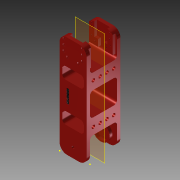
# Autodesk Inventor part: 150mm Link
Saved by Autodesk Inventor 2015 (Build 190159000, 159)
## iProperties
Created: 2016-11-30
Part Number: 150mm Link
Material: Generic
Document SubType Name: Modeling
Designer: Rudge-Top
Density: 1 g/cm^3
Appearance: Orange-Red
Author: Rudge-Top
Autodesk Inventor part; units mm, degrees
ref_plane "YZ Plane" through (0, 0, 0) normal (1, 0, 0) x (0, 1, 0)
ref_plane "XZ Plane" through (0, 0, 0) normal (0, 1, 0) x (-1, 0, 0)
ref_plane "XY Plane" through (0, 0, 0) normal (0, 0, 1) x (1, 0, 0)
sketch "Sketch1" plane through (0, 0, 0) normal (1, 0, 0) x (0, 1, 0)
  line L0 (120, 0) -> (150, 0)
  line L1 (150, 0) -> (150, -40)
  line L2 (150, -40) -> (120, -40)
  line L3 (150, 5) -> (0, 5)
  line L4 (0, -45) -> (150, -45)
  line L5 (150, 0) -> (150, 5)
  line L6 (150, -40) -> (150, -45)
  line L7 (0, -40) -> (0, -45)
  line L8 (0, 0) -> (0, 5)
  line L9 (115, -5) -> (115, -35)
  arc A0 (120, 0) -> (115, -5) centre (120, -5) ccw
  arc A1 (115, -35) -> (120, -40) centre (120, -35) ccw
  line L10 (87.5, 0) -> (62.5, 0)
  line L11 (57.5, -5) -> (57.5, -35)
  line L12 (62.5, -40) -> (87.5, -40)
  line L13 (92.5, -35) -> (92.5, -5)
  arc A2 (87.5, -40) -> (92.5, -35) centre (87.5, -35) ccw
  arc A3 (57.5, -35) -> (62.5, -40) centre (62.5, -35) ccw
  arc A4 (62.5, 0) -> (57.5, -5) centre (62.5, -5) ccw
  arc A5 (92.5, -5) -> (87.5, 0) centre (87.5, -5) ccw
  line L14 (0, 0) -> (30, 0)
  line L15 (35, -5) -> (35, -35)
  line L16 (30, -40) -> (0, -40)
  arc A6 (35, -5) -> (30, 0) centre (30, -5) ccw
  arc A7 (30, -40) -> (35, -35) centre (30, -35) ccw
  point P0 (57.5, -40)
  point P1 (92.5, -40)
  point P2 (35, 0)
  dimension "d1" = 150
  dimension "d2" = 40
  dimension "d3" = 90
  dimension "d4" = 5
  dimension "d5" = 35
  dimension "d6" = 5
  dimension "d7" = 35
  dimension "d8" = 5
  dimension "d9" = 22.5
  dimension "d10" = 5
  dimension "d11" = 35
  dimension "d12" = 5
  constraints: 34 end point, 16 point on circle, 16 tangent, 9 point on line, 8 centre point, 8 perpendicular, 5 equal radius, 3 horizontal, 2 parallel
  measures "d1" distance of L8.start L0.end
  measures "d2" distance of L0.end L1.end
  measures "d3" angle of L0 L1
  measures "d4" distance between parallel lines of L0 L3
  measures "d5" distance between parallel lines of L1 L9
  measures "d6" radius of A0
  measures "d7" distance of point (92.5, -40) point (57.5, -40)
  measures "d8" distance between parallel lines of L3 L10
  measures "d9" distance between parallel lines of L13 L9
  measures "d10" radius of A2
  measures "d11" distance of L8.start point (35, 0)
  measures "d12" radius of A6
extrude "Extrusion1" add sketch "Sketch1" along normal blind 40 contours A0 L9 A1 L2 L6 L4 L7 L16 A7 L15 A6 L14 L8 L3 L5 L0
sketch "Sketch2" plane through (40, 0, 0) normal (1, 0, 0) x (0, 0, -1)
  arc A0 (35, 57.5) -> (40, 62.5) centre (35, 62.5) ccw projected
  line L0 (35, 57.5) -> (5, 57.5) projected
  arc A1 (0, 62.5) -> (5, 57.5) centre (5, 62.5) ccw projected
  line L1 (0, 62.5) -> (0, 87.5) projected
  arc A2 (5, 92.5) -> (0, 87.5) centre (5, 87.5) ccw projected
  line L2 (5, 92.5) -> (35, 92.5) projected
  arc A3 (40, 87.5) -> (35, 92.5) centre (35, 87.5) ccw projected
  line L3 (40, 87.5) -> (40, 62.5) projected
  line L4 (0, 0) -> (0, 30) projected
  arc A4 (5, 35) -> (0, 30) centre (5, 30) ccw projected
  line L5 (5, 35) -> (35, 35) projected
  arc A5 (40, 30) -> (35, 35) centre (35, 30) ccw projected
  line L6 (40, 30) -> (40, 0) projected
  line L7 (40, 0) -> (45, 0) projected
  line L8 (45, 0) -> (45, 150) projected
  line L9 (45, 150) -> (40, 150) projected
  line L10 (40, 150) -> (40, 120) projected
  arc A6 (35, 115) -> (40, 120) centre (35, 120) ccw projected
  line L11 (35, 115) -> (5, 115) projected
  arc A7 (0, 120) -> (5, 115) centre (5, 120) ccw projected
  line L12 (0, 120) -> (0, 150) projected
  line L13 (0, 150) -> (-5, 150) projected
  line L14 (-5, 150) -> (-5, 0) projected
  line L15 (-5, 0) -> (0, 0) projected
  circle A8 centre (35, 45.25) radius 2.5
  circle A9 centre (25, 45.25) radius 2.5
  circle A10 centre (15, 45.25) radius 2.5
  circle A11 centre (5, 45.25) radius 2.5
  circle A12 centre (35, 104.75) radius 2.5
  circle A13 centre (25, 104.75) radius 2.5
  circle A14 centre (15, 104.75) radius 2.5
  circle A15 centre (5, 104.75) radius 2.5
  dimension "d15" = 5
  dimension "d16" = 5
  dimension "d17" = 5
  dimension "d18" = 5
  dimension "d19" = 10
  dimension "d20" = 20
  dimension "d21" = 30
  dimension "d22" = 40
  dimension "d23" = 5
  dimension "d24" = 5
  dimension "d25" = 5
  dimension "d26" = 5
  dimension "d27" = 12.25
  dimension "d28" = 12.25
  dimension "d29" = 12.25
  dimension "d30" = 12.25
  dimension "d31" = 12.25
  dimension "d32" = 12.25
  dimension "d33" = 12.25
  dimension "d34" = 12.25
  constraints: 8 centre point
  measures "d15" diameter of A8
  measures "d16" diameter of A9
  measures "d17" diameter of A10
  measures "d18" diameter of A11
  measures "d19" distance from line of L14 A11.centre
  measures "d20" distance from line of A10.centre L14
  measures "d21" distance from line of A9.centre L14
  measures "d22" distance from line of A8.centre L14
  measures "d23" diameter of A12
  measures "d24" diameter of A13
  measures "d25" diameter of A14
  measures "d26" diameter of A15
  measures "d27" distance from line of A12.centre L2
  measures "d28" distance from line of L2 A13.centre
  measures "d29" distance from line of L2 A14.centre
  measures "d30" distance from line of L2 A15.centre
  measures "d31" distance from line of A8.centre L0
  measures "d32" distance from line of A9.centre L0
  measures "d33" distance from line of A10.centre L0
  measures "d34" distance from line of A11.centre L0
extrude "Extrusion2" cut sketch "Sketch2" against normal blind 25 contours A8 | A9 | A10 | A11 | A12 | A13 | A14 | A15
fillet "Fillet1" radius 11 8 edges at (40, 0, 2.5) (0, 0, 2.5) (40, 0, -42.5) (0, 0, -42.5) (40, 150, 2.5) (40, 150, -42.5) (0, 150, -42.5) (0, 150, 2.5)
sketch "Sketch3" plane through (0, 11, -45) normal (0, 0, -1) x (-1, 0, 0)
  line L0 (0, 51.5) -> (-40, 51.5) projected
  arc A0 (0, 128) -> (-11, 139) centre (-11, 128) ccw projected
  line L1 (-11, 139) -> (-29, 139) projected
  arc A1 (-29, 139) -> (-40, 128) centre (-29, 128) ccw projected
  line L2 (-40, 0) -> (-40, 128) projected
  arc A2 (-40, 0) -> (-29, -11) centre (-29, 0) ccw projected
  line L3 (-11, -11) -> (-29, -11) projected
  arc A3 (-11, -11) -> (0, 0) centre (-11, 0) ccw projected
  line L4 (0, 0) -> (0, 128) projected
  line L5 (-40, 51.5) -> (-40, 46.5) projected
  line L6 (-40, 46.5) -> (-40, 51.5) projected
  line L7 (-40, 51.5) -> (-40, 76.5) projected
  line L8 (-40, 76.5) -> (-40, 81.5) projected
  line L9 (-40, 81.5) -> (-40, 76.5) projected
  line L10 (-40, 76.5) -> (-40, 51.5) projected
  line L11 (-40, 91.25) -> (-40, 96.25) projected
  line L12 (-40, 91.25) -> (-40, 96.25) projected
  line L13 (-40, 31.75) -> (-40, 36.75) projected
  line L14 (-40, 31.75) -> (-40, 36.75) projected
  line L15 (-40, 31.75) -> (-40, 36.75) projected
  line L16 (-40, 31.75) -> (-40, 36.75) projected
  line L17 (-40, 91.25) -> (-40, 96.25) projected
  line L18 (-40, 91.25) -> (-40, 96.25) projected
  line L19 (-40, 128) -> (-40, 109) projected
  line L20 (-40, 109) -> (-40, 104) projected
  line L21 (-40, 104) -> (-40, 109) projected
  line L22 (-40, 109) -> (-40, 128) projected
  line L23 (-40, 128) -> (-40, 0) projected
  line L24 (-40, 0) -> (-40, 19) projected
  line L25 (-40, 19) -> (-40, 24) projected
  line L26 (-40, 24) -> (-40, 19) projected
  line L27 (-40, 19) -> (-40, 0) projected
  line L28 (-40, 0) -> (-40, 128) projected
  line L29 (-9, 26.5) -> (-31, 26.5)
  line L30 (-36, 31.5) -> (-36, 39)
  line L31 (-31, 44) -> (-9, 44)
  line L32 (-4, 39) -> (-4, 31.5)
  arc A4 (-36, 31.5) -> (-31, 26.5) centre (-31, 31.5) ccw
  arc A5 (-31, 44) -> (-36, 39) centre (-31, 39) ccw
  arc A6 (-4, 39) -> (-9, 44) centre (-9, 39) ccw
  arc A7 (-9, 26.5) -> (-4, 31.5) centre (-9, 31.5) ccw
  line L33 (-9, 84) -> (-31, 84)
  line L34 (-36, 89) -> (-36, 96.5)
  line L35 (-31, 101.5) -> (-9, 101.5)
  line L36 (-4, 96.5) -> (-4, 89)
  arc A8 (-36, 89) -> (-31, 84) centre (-31, 89) ccw
  arc A9 (-31, 101.5) -> (-36, 96.5) centre (-31, 96.5) ccw
  arc A10 (-4, 96.5) -> (-9, 101.5) centre (-9, 96.5) ccw
  arc A11 (-9, 84) -> (-4, 89) centre (-9, 89) ccw
  point P0 (0, -11)
  point P1 (-36, 44)
  point P2 (-36, 26.5)
  point P3 (-4, 44)
  dimension "d38" = 32
  dimension "d39" = 17.5
  dimension "d40" = 55
  dimension "d41" = 5
  dimension "d42" = 5
  dimension "d43" = 55
  dimension "d73" = 4
  dimension "d74" = 4
  dimension "d75" = 32
  constraints: 16 end point, 16 point on circle, 16 tangent, 8 centre point, 6 equal radius, 6 point on line, 4 parallel, 2 horizontal, 2 perpendicular
  measures "d38" distance of point (-36, 44) point (-4, 44)
  measures "d39" distance of point (-36, 26.5) point (-36, 44)
  measures "d40" distance between parallel lines of L3 L31
  measures "d41" radius of A4
  measures "d42" radius of A8
  measures "d43" distance between parallel lines of L1 L33
  measures "d73" distance between parallel lines of L4 L32
  measures "d74" distance between parallel lines of L4 L36
  measures "d75" distance between parallel lines of L36 L34
extrude "Extrusion3" cut sketch "Sketch3" against normal blind 100 contours L29 A4 L30 A5 L31 A6 L32 A7 | L33 A8 L34 A9 L35 A10 L36 A11
sketch "Sketch4" plane through (0, 11, 5) normal (0, 0, 1) x (1, 0, 0)
  line L0 (13.751451, 74.450189) -> (13.751451, 54.540799) construction
  line L1 (13.751451, 54.540799) -> (10.190186, 54.540799) construction
  line L2 (10.190186, 54.540799) -> (10.190186, 74.450189) construction
  line L3 (10.190186, 74.450189) -> (13.751451, 74.450189) construction
  point P0 (0, -11)
  constraints: 2 other
sketch "Sketch5" plane through (40, 0, 0) normal (1, 0, 0) x (0, 0, -1)
  point P0 (0, 0)
sketch "Sketch6" plane through (0, 30, -40) normal (0, 0, 1) x (1, 0, 0)
  arc A0 (0, -19) -> (11, -30) centre (11, -19) ccw
  line L0 (11, -30) -> (29, -30)
  arc A1 (29, -30) -> (40, -19) centre (29, -19) ccw
  line L1 (40, 0) -> (40, -19)
  line L2 (0, 0) -> (40, 0)
  line L3 (0, 0) -> (0, -19)
  arc A2 (12.000009, -23.549844) -> (12.000009, -8.450156) centre (20, -16) ccw
  line L4 (12.000009, -34.540496) -> (12.000009, 2.540496)
  arc A3 (12.000009, -26.246958) -> (12.000009, -5.753042) centre (20, -16) ccw
  point P0 (0, -30)
  point P1 (12.000009, -16.011855)
  point P2 (20.011855, -23.999991)
  point P3 (27.999991, -15.988145)
  point P4 (19.988145, -8.000009)
  dimension "d46" = 22
  dimension "d47" = 14
  dimension "d48" = 8
  dimension "d51" = 360
  dimension "d71" = 20
  dimension "d115" = 13
  constraints: 5 point on line, 4 point on circle, 2 centre point, 2 end point, 1 coincident, 1 vertical, 5 other
  measures "d46" diameter of A2
  measures "d47" distance from line of L0 A2.centre
  measures "d48" distance of A2.centre point (12, -16.012)
  measures "d71" distance from line of L3 A2.centre
  measures "d115" radius of A3
hole "Hole1" at (20.011855, 6.000009, -40) at (12.000009, 13.988145, -40) at (27.999991, 14.011855, -40) at (19.988145, 21.999991, -40) direction (0, 0, -1) diameter 2 end through all
extrude "Extrusion4" add sketch "Sketch6" along normal blind 4 contours L4 A2 A3
sketch "Sketch7" plane through (0, 11, 5) normal (0, 0, 1) x (1, 0, 0)
  arc A0 (4, 31.5) -> (9, 26.5) centre (9, 31.5) ccw
  line L0 (4, 31.5) -> (4, 39)
  arc A1 (9, 44) -> (4, 39) centre (9, 39) ccw
  line L1 (9, 44) -> (31, 44)
  arc A2 (36, 39) -> (31, 44) centre (31, 39) ccw
  line L2 (36, 39) -> (36, 31.5)
  arc A3 (31, 26.5) -> (36, 31.5) centre (31, 31.5) ccw
  line L3 (31, 26.5) -> (9, 26.5)
  arc A4 (31, 84) -> (36, 89) centre (31, 89) ccw
  line L4 (31, 84) -> (9, 84)
  arc A5 (4, 89) -> (9, 84) centre (9, 89) ccw
  line L5 (4, 89) -> (4, 96.5)
  arc A6 (9, 101.5) -> (4, 96.5) centre (9, 96.5) ccw
  line L6 (9, 101.5) -> (31, 101.5)
  arc A7 (36, 96.5) -> (31, 101.5) centre (31, 96.5) ccw
  line L7 (36, 96.5) -> (36, 89)
  arc A8 (11, 139) -> (0, 128) centre (11, 128) ccw
  line L8 (0, 128) -> (0, 0)
  arc A9 (0, 0) -> (11, -11) centre (11, 0) ccw
  line L9 (11, -11) -> (29, -11)
  arc A10 (29, -11) -> (40, 0) centre (29, 0) ccw
  line L10 (40, 128) -> (40, 0)
  arc A11 (40, 128) -> (29, 139) centre (29, 128) ccw
  line L11 (11, 139) -> (29, 139)
  circle A12 centre (27.999991, 3.011855) radius 1
  circle A13 centre (19.988145, 10.999991) radius 1
  circle A14 centre (12.000009, 2.988145) radius 1
  circle A15 centre (20.011855, -4.999991) radius 1
  point P0 (0, -11)
  point P1 (20, 2.999991)
  dimension "d63" = 8
  dimension "d72" = 8
  measures "d63" distance of point (20, 3) A12.centre
  measures "d72" distance of A13.centre point (20, 3)
hole "Hole2" at (20, 13.999991, 5) direction (0, 0, -1) diameter 4 end through all
sketch "Sketch8" plane through (0, 120, -40) normal (0, 0, 1) x (1, 0, 0)
  arc A0 (11, 30) -> (0, 19) centre (11, 19) ccw
  line L0 (0, 19) -> (0, 0)
  line L1 (0, 0) -> (40, 0)
  line L2 (40, 19) -> (40, 0)
  arc A1 (40, 19) -> (29, 30) centre (29, 19) ccw
  line L3 (11, 30) -> (29, 30)
  line L4 (11, 30) -> (29, 30)
  line L5 (20, 10) -> (20, 0)
  line L6 (29, 30) -> (29.5, 30)
  arc A2 (40, 19) -> (29, 30) centre (29, 19) ccw
  line L7 (29.5, 30) -> (29.5, 10)
  line L8 (29.5, 10) -> (24, 10)
  line L9 (0, 0) -> (40, 0)
  line L10 (37.5, 0) -> (37.5, 25.98212)
  arc A3 (37.5, 25.98212) -> (29.5, 30) centre (28.954916, 18.941344) ccw
  line L11 (24, 10) -> (24, 0)
  arc A4 (11, 30) -> (0, 19) centre (11, 19) ccw
  line L12 (10.5, 30) -> (10.5, 10)
  line L13 (10.5, 10) -> (16, 10)
  line L14 (2.5, 0) -> (2.5, 25.98212)
  arc A5 (10.5, 30) -> (2.5, 25.98212) centre (11.045084, 18.941344) ccw
  line L15 (16, 10) -> (16, 0)
  line L16 (37.5, 0) -> (24, 0)
  line L17 (31, -7.5) -> (9, -7.5)
  line L18 (16, 0) -> (2.5, 0)
  arc A6 (10.5, 30) -> (2.5, 25.98212) centre (11.045084, 18.941344) ccw
  point P0 (0, -120)
  dimension "d77" = 10
  dimension "d78" = 9.5
  dimension "d80" = 17.5
  dimension "d81" = 4
  constraints: 24 end point, 9 point on circle, 8 symmetric about line, 4 centre point, 3 point on line, 3 vertical, 2 tangent, 1 collinear, 1 midpoint, 1 parallel, 1 perpendicular, 2 other
  measures "d77" distance between parallel lines of L8 L1
  measures "d78" distance between parallel lines of L5 L7
  measures "d80" distance between parallel lines of L10 L5
  measures "d81" distance between parallel lines of L5 L11
sketch "Sketch8 outline for Extrusion5" plane through (0, 120, -40) normal (0, 0, 1) x (1, 0, 0)
  line L0 (37.5, 0) -> (37.5, 25.98212)
  line L1 (24, 0) -> (37.5, 0)
  line L2 (24, 10) -> (24, 0)
  line L3 (29.5, 10) -> (24, 10)
  line L4 (29.5, 30) -> (29.5, 10)
  arc A0 (37.5, 25.98212) -> (29.5, 30) centre (28.954916, 18.941344) ccw
  line L5 (2.5, 25.98212) -> (2.5, 0)
  arc A1 (10.5, 30) -> (2.5, 25.98212) centre (11.045084, 18.941344) ccw
  line L6 (10.5, 10) -> (10.5, 30)
  line L7 (16, 10) -> (10.5, 10)
  line L8 (16, 0) -> (16, 10)
  line L9 (2.5, 0) -> (16, 0)
extrude "Extrusion5" add sketch "Sketch8 outline for Extrusion5" along normal blind 4
ref_plane "Work Plane1" through (0, 11, -20) normal (0, 0, 1) x (1, 0, 0)
mirror "Mirror1" about plane through (0, 11, -20) normal (0, 0, 1) of "Extrusion5"
sketch "Sketch9" plane through (0, 11, -45) normal (0, 0, -1) x (-1, 0, 0)
  circle A0 centre (-20, 2.999991) radius 2
  circle A1 centre (-27.999991, 3.011855) radius 1
  circle A2 centre (-20.011855, -4.999991) radius 1
  circle A3 centre (-12.000009, 2.988145) radius 1
  circle A4 centre (-19.988145, 10.999991) radius 1
  arc A5 (-9, 26.5) -> (-4, 31.5) centre (-9, 31.5) ccw
  line L0 (-9, 26.5) -> (-31, 26.5)
  arc A6 (-36, 31.5) -> (-31, 26.5) centre (-31, 31.5) ccw
  line L1 (-36, 31.5) -> (-36, 39)
  arc A7 (-31, 44) -> (-36, 39) centre (-31, 39) ccw
  line L2 (-31, 44) -> (-9, 44)
  arc A8 (-4, 39) -> (-9, 44) centre (-9, 39) ccw
  line L3 (-4, 39) -> (-4, 31.5)
  arc A9 (-36, 89) -> (-31, 84) centre (-31, 89) ccw
  line L4 (-36, 89) -> (-36, 96.5)
  arc A10 (-31, 101.5) -> (-36, 96.5) centre (-31, 96.5) ccw
  line L5 (-31, 101.5) -> (-9, 101.5)
  arc A11 (-4, 96.5) -> (-9, 101.5) centre (-9, 96.5) ccw
  line L6 (-4, 96.5) -> (-4, 89)
  arc A12 (-9, 84) -> (-4, 89) centre (-9, 89) ccw
  line L7 (-9, 84) -> (-31, 84)
  arc A13 (0, 128) -> (-11, 139) centre (-11, 128) ccw
  line L8 (-11, 139) -> (-29, 139)
  arc A14 (-29, 139) -> (-40, 128) centre (-29, 128) ccw
  line L9 (-40, 0) -> (-40, 128)
  arc A15 (-40, 0) -> (-29, -11) centre (-29, 0) ccw
  line L10 (-11, -11) -> (-29, -11)
  arc A16 (-11, -11) -> (0, 0) centre (-11, 0) ccw
  line L11 (0, 0) -> (0, 128)
  arc A17 (-29.5, 139) -> (-37.5, 134.98212) centre (-28.954916, 127.941344) ccw
  line L12 (-37.5, 109) -> (-37.5, 134.98212)
  line L13 (-24, 109) -> (-37.5, 109)
  line L14 (-24, 119) -> (-24, 109)
  line L15 (-29.5, 119) -> (-24, 119)
  line L16 (-29.5, 139) -> (-29.5, 119)
  line L17 (-2.5, 109) -> (-16, 109)
  line L18 (-2.5, 134.98212) -> (-2.5, 109)
  arc A18 (-2.5, 134.98212) -> (-10.5, 139) centre (-11.045084, 127.941344) ccw
  line L19 (-10.5, 119) -> (-10.5, 139)
  line L20 (-16, 119) -> (-10.5, 119)
  line L21 (-16, 109) -> (-16, 119)
  line L22 (-16, 109) -> (-24, 109)
  line L23 (-20, 109) -> (-20, 113.032959)
  point P0 (0, -11)
  point P1 (-28, 114)
  point P2 (-12, 114)
  point P3 (-6.5, 119.25)
  point P4 (-6.5, 127.25)
  point P5 (-6.5, 135.25)
  point P6 (-33.5, 119.25)
  point P7 (-33.5, 127.25)
  point P8 (-33.5, 135.25)
  dimension "d84" = 4
  dimension "d85" = 16
  dimension "d86" = 5
  dimension "d87" = 5.25
  dimension "d88" = 8
  dimension "d89" = 8
  dimension "d90" = 4
  dimension "d91" = 4
  dimension "d92" = 4
  constraints: 4 end point, 3 symmetric about line, 1 horizontal, 1 midpoint, 1 vertical
  measures "d84" distance from line of L14 point (-28, 114)
  measures "d85" distance of point (-12, 114) point (-28, 114)
  measures "d86" distance from line of point (-28, 114) L13
  measures "d87" vertical distance of point (-12, 114) point (-6.5, 119.25)
  measures "d88" distance of point (-6.5, 127.25) point (-6.5, 119.25)
  measures "d89" distance of point (-6.5, 127.25) point (-6.5, 135.25)
  measures "d90" distance from line of L18 point (-6.5, 119.25)
  measures "d91" distance from line of L18 point (-6.5, 127.25)
  measures "d92" distance from line of L18 point (-6.5, 135.25)
hole "Hole3" at (33.5, 146.25, -45) at (33.5, 138.25, -45) at (33.5, 130.25, -45) at (28, 125, -45) at (12, 125, -45) at (6.5, 130.25, -45) at (6.5, 138.25, -45) at (6.5, 146.25, -45) direction (0, 0, 1) diameter 2 end through all
sketch "Sketch10" plane through (0, 11, 5) normal (0, 0, 1) x (1, 0, 0)
  circle A0 centre (6.5, 127.25) radius 1
  circle A1 centre (12, 114) radius 1
  circle A2 centre (33.5, 119.25) radius 1
  circle A3 centre (33.5, 135.25) radius 1
  circle A4 centre (33.5, 127.25) radius 1
  circle A5 centre (28, 114) radius 1
  circle A6 centre (6.5, 119.25) radius 1
  circle A7 centre (6.5, 135.25) radius 1
  circle A8 centre (20, 2.999991) radius 2
  arc A9 (4, 31.5) -> (9, 26.5) centre (9, 31.5) ccw
  line L0 (4, 31.5) -> (4, 39)
  arc A10 (9, 44) -> (4, 39) centre (9, 39) ccw
  line L1 (9, 44) -> (31, 44)
  arc A11 (36, 39) -> (31, 44) centre (31, 39) ccw
  line L2 (36, 39) -> (36, 31.5)
  arc A12 (31, 26.5) -> (36, 31.5) centre (31, 31.5) ccw
  line L3 (31, 26.5) -> (9, 26.5)
  arc A13 (31, 84) -> (36, 89) centre (31, 89) ccw
  line L4 (31, 84) -> (9, 84)
  arc A14 (4, 89) -> (9, 84) centre (9, 89) ccw
  line L5 (4, 89) -> (4, 96.5)
  arc A15 (9, 101.5) -> (4, 96.5) centre (9, 96.5) ccw
  line L6 (9, 101.5) -> (31, 101.5)
  arc A16 (36, 96.5) -> (31, 101.5) centre (31, 96.5) ccw
  line L7 (36, 96.5) -> (36, 89)
  arc A17 (11, 139) -> (0, 128) centre (11, 128) ccw
  line L8 (0, 128) -> (0, 0)
  arc A18 (0, 0) -> (11, -11) centre (11, 0) ccw
  line L9 (11, -11) -> (29, -11)
  arc A19 (29, -11) -> (40, 0) centre (29, 0) ccw
  line L10 (40, 128) -> (40, 0)
  arc A20 (40, 128) -> (29, 139) centre (29, 128) ccw
  line L11 (11, 139) -> (29, 139)
  line L12 (28, 111.690599) -> (26, 112.845299)
  line L13 (26, 112.845299) -> (26, 115.154701)
  line L14 (26, 115.154701) -> (28, 116.309401)
  line L15 (28, 116.309401) -> (30, 115.154701)
  line L16 (30, 115.154701) -> (30, 112.845299)
  line L17 (30, 112.845299) -> (28, 111.690599)
  line L18 (12, 111.690599) -> (10, 112.845299)
  line L19 (10, 112.845299) -> (10, 115.154701)
  line L20 (10, 115.154701) -> (12, 116.309401)
  line L21 (12, 116.309401) -> (14, 115.154701)
  line L22 (14, 115.154701) -> (14, 112.845299)
  line L23 (14, 112.845299) -> (12, 111.690599)
  line L24 (6.5, 116.940599) -> (4.5, 118.095299)
  line L25 (4.5, 118.095299) -> (4.5, 120.404701)
  line L26 (4.5, 120.404701) -> (6.5, 121.559401)
  line L27 (6.5, 121.559401) -> (8.5, 120.404701)
  line L28 (8.5, 120.404701) -> (8.5, 118.095299)
  line L29 (8.5, 118.095299) -> (6.5, 116.940599)
  line L30 (6.5, 124.940599) -> (4.5, 126.095299)
  line L31 (4.5, 126.095299) -> (4.5, 128.404701)
  line L32 (4.5, 128.404701) -> (6.5, 129.559401)
  line L33 (6.5, 129.559401) -> (8.5, 128.404701)
  line L34 (8.5, 128.404701) -> (8.5, 126.095299)
  line L35 (8.5, 126.095299) -> (6.5, 124.940599)
  circle A21 centre (6.5, 127.25) radius 1
  circle A22 centre (6.5, 119.25) radius 1
  circle A23 centre (12, 114) radius 1
  circle A24 centre (28, 114) radius 1
  line L36 (33.5, 132.940599) -> (31.5, 134.095299)
  line L37 (31.5, 134.095299) -> (31.5, 136.404701)
  line L38 (31.5, 136.404701) -> (33.5, 137.559401)
  line L39 (33.5, 137.559401) -> (35.5, 136.404701)
  line L40 (35.5, 136.404701) -> (35.5, 134.095299)
  line L41 (35.5, 134.095299) -> (33.5, 132.940599)
  line L42 (6.5, 137.559401) -> (8.5, 136.404701)
  line L43 (8.5, 136.404701) -> (8.5, 134.095299)
  line L44 (8.5, 134.095299) -> (6.5, 132.940599)
  line L45 (6.5, 132.940599) -> (4.5, 134.095299)
  line L46 (4.5, 134.095299) -> (4.5, 136.404701)
  line L47 (4.5, 136.404701) -> (6.5, 137.559401)
  circle A25 centre (6.5, 135.25) radius 1
  circle A26 centre (33.5, 135.25) radius 1
  line L48 (33.5, 129.559401) -> (35.5, 128.404701)
  line L49 (35.5, 128.404701) -> (35.5, 126.095299)
  line L50 (35.5, 126.095299) -> (33.5, 124.940599)
  line L51 (33.5, 124.940599) -> (31.5, 126.095299)
  line L52 (31.5, 126.095299) -> (31.5, 128.404701)
  line L53 (31.5, 128.404701) -> (33.5, 129.559401)
  line L54 (33.5, 121.559401) -> (35.5, 120.404701)
  line L55 (35.5, 120.404701) -> (35.5, 118.095299)
  line L56 (35.5, 118.095299) -> (33.5, 116.940599)
  line L57 (33.5, 116.940599) -> (31.5, 118.095299)
  line L58 (31.5, 118.095299) -> (31.5, 120.404701)
  line L59 (31.5, 120.404701) -> (33.5, 121.559401)
  circle A27 centre (33.5, 127.25) radius 1
  circle A28 centre (33.5, 119.25) radius 1
  point P0 (0, -11)
  dimension "d102" = 4
  dimension "d103" = 4
  dimension "d104" = 4
  dimension "d105" = 4
  dimension "d111" = 4
  dimension "d112" = 4
  dimension "d113" = 4
  dimension "d114" = 4
  constraints: 96 end point, 8 centre point, 7 coincident, 3 concentric, 52 other
  measures "d102" distance between parallel lines of L16 L13
  measures "d103" distance between parallel lines of L22 L19
  measures "d104" distance between parallel lines of L28 L25
  measures "d105" distance between parallel lines of L34 L31
  measures "d111" distance between parallel lines of L37 L40
  measures "d112" distance between parallel lines of L43 L46
  measures "d113" distance between parallel lines of L55 L58
  measures "d114" distance between parallel lines of L49 L52
extrude "Extrusion6" cut sketch "Sketch10" against normal blind 1.6 contours L12 L13 L14 L15 L16 L17 | L18 L19 L20 L21 L22 L23 | L24 L25 L26 L27 L28 L29 | L30 L31 L32 L33 L34 L35 | L36 L37 L38 L39 L40 L41 | L42 L43 L44 L45 L46 L47 | L48 L49 L50 L51 L52 L53 | L54 L55 L56 L57 L58 L59
mirror "Mirror2" about plane through (0, 11, -20) normal (0, 0, 1) of "Extrusion6"
sketch "Sketch11" plane through (40, 0, 0) normal (1, 0, 0) x (0, 0, -1)
  point P0 (0, 0)
body "Solid1"
